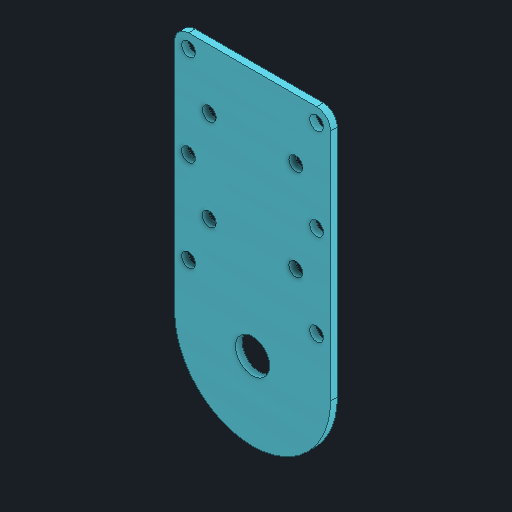
# Autodesk Inventor part: femur_outside_steel
Saved by Autodesk Inventor 2026 (Build 300175000, 175)
## iProperties
Created: 2026-04-25
Part Number: femur_outside_steel
Material: Сталь
Document SubType Name: Modeling
Designer: user
Density: 7.85 g/cm^3
Appearance: Серо-синий
Mass: 207.185 g
Surface Area: 195.364 cm^2
Volume: 26.393 cm^3
Author: user
Autodesk Inventor part; units mm, degrees
ref_plane "YZ Plane" through (0, 0, 0) normal (1, 0, 0) x (0, 1, 0)
ref_plane "XZ Plane" through (0, 0, 0) normal (0, 1, 0) x (-1, 0, 0)
ref_plane "XY Plane" through (0, 0, 0) normal (0, 0, 1) x (1, 0, 0)
sketch "Эскиз3" plane through (0, 0, 0) normal (0, 0, 1) x (1, 0, 0)
  line L0 (110.155, -68.7957) -> (60.155, -68.7957) construction
  line L1 (60.155, -68.7957) -> (60.155, 68.0464) construction
  line L2 (110.155, 68.0464) -> (110.155, -68.7957) construction
  circle A0 centre (57.105, -53.7957) radius 3.05
  circle A1 centre (57.105, -13.7957) radius 3.05
  circle A2 centre (57.105, 26.2043) radius 3.05
  circle A3 centre (113.205, -53.7957) radius 3.05
  circle A4 centre (113.205, -13.7957) radius 3.05
  circle A5 centre (113.205, 26.2043) radius 3.05
  circle A6 centre (85.155, -76.2957) radius 7.5
  line L3 (85.155, -21.4404) -> (85.155, -113.936) construction
  arc A7 (119.305, 26.2043) -> (113.205, 32.3043) centre (113.205, 26.2043) ccw
  arc A8 (57.105, 32.3043) -> (51.005, 26.2043) centre (57.105, 26.2043) ccw
  line L4 (113.205, 32.3043) -> (57.105, 32.3043)
  line L5 (119.305, 26.2043) -> (119.305, -76.2957)
  line L6 (51.005, 26.2043) -> (51.005, -76.2957)
  arc A9 (51.005, -76.2957) -> (119.305, -76.2957) centre (85.155, -76.2957) ccw
  circle A10 centre (66.205, -33.7957) radius 3.05
  circle A11 centre (66.205, 6.2043) radius 3.05
  circle A12 centre (104.105, -33.7957) radius 3.05
  circle A13 centre (104.105, 6.2043) radius 3.05
  point P0 (0, 0)
  dimension "d8" = 50
  dimension "d11" = 40
  dimension "d14" = 56.1
  dimension "d17" = 6.1
  dimension "d18" = 15
  dimension "d19" = 15
  dimension "d20" = 12.2
  dimension "d21" = 12.2
  dimension "d24" = 40
  dimension "d27" = 37.9
  dimension "d30" = 20
  constraints: 14 centre point, 14 end point, 6 point on circle, 6 tangent, 4 vertical, 3 coincident, 3 horizontal, 2 perpendicular, 1 equal radius, 1 horizontal alignment, 1 parallel, 1 point on line, 1 symmetric about line, 18 other
  measures "d8" distance of L0.start L0.end
  measures "d11" distance of A0.centre A1.centre
  measures "d14" distance of A0.centre A3.centre
  measures "d17" diameter of A0
  measures "d18" distance from line of L0 A3.centre
  measures "d19" diameter of A6
  measures "d20" diameter of A7
  measures "d21" diameter of A8
  measures "d24" distance of A10.centre A11.centre
  measures "d27" distance of A10.centre A12.centre
  measures "d30" vertical distance of A3.centre A12.centre
extrude "Выдавливание3" add sketch "Эскиз3" along normal blind 3
equation "\"d8\" = hight_profile_femur"
equation "\"d14\" = hight_profile_femur + d_main_screw_holes"
equation "\"d17\" = d_main_screw_holes"
equation "\"d19\" = d_main_shaft"
equation "\"d20\" = 2 * d_main_screw_holes"
equation "\"d21\" = 2 * d_main_screw_holes"
equation "\"d27\" = -d_main_screw_holes + hight_profile_femur - 2 * thickness_profile_femur"
equation "\"d6\" = thickness_steel"
equation "\"tolerance_plazma\" = 0.1"
equation "\"thickness_steel\" = 3"
equation "\"d_main_screw_holes\" = 6.1"
equation "\"d_main_shaft\" = 15"
equation "\"thickness_profile_tibea\" = 3"
equation "\"hight_shaft_shift\" = 37"
equation "\"thickness_profile_femur\" = 3"
equation "\"width_shaft_shift\" = 35"
equation "\"hight_profile_femur\" = 50"
equation "\"width_flattened_surface\" = 12"
